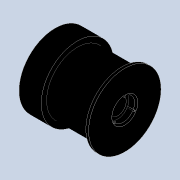
# Autodesk Inventor part: 8mm ID 15mm Deep Idler Pully
Saved by Autodesk Inventor 2022 (Build 260153000, 153)
## iProperties
Created: 2021-10-11
Part Number: 8mm ID 15mm Deep Idler Pully
Material: Generic
Document SubType Name: Modeling
Designer: Coy
Density: 1 g/cm^3
Appearance: Anodized - Black
Author: Coy
Autodesk Inventor part; units mm, degrees
ref_plane "YZ Plane" through (0, 0, 0) normal (1, 0, 0) x (0, 1, 0)
ref_plane "XZ Plane" through (0, 0, 0) normal (0, 1, 0) x (-1, 0, 0)
ref_plane "XY Plane" through (0, 0, 0) normal (0, 0, 1) x (1, 0, 0)
sketch "Sketch1" plane through (0, 0, 0) normal (1, 0, 0) x (0, 1, 0)
  circle A0 centre (0, 0) radius 4
  circle A1 centre (0, 0) radius 13
  dimension "d0" = 8
  dimension "d1" = 26
  constraints: 2 centre point, 2 coincident
  measures "d0" diameter of A0
  measures "d1" diameter of A1
extrude "Extrusion1" add sketch "Sketch1" along normal blind 2.5
sketch "Sketch2" plane through (2.5, 0, 0) normal (1, 0, 0) x (0, 0, -1)
  circle A0 centre (0, 0) radius 3
  circle A1 centre (0, 0) radius 13
  dimension "d4" = 6
  constraints: 2 centre point, 2 coincident
  measures "d4" diameter of A0
extrude "Extrusion2" add sketch "Sketch2" along normal blind 5.5
sketch "Sketch3" plane through (8, 0, 0) normal (1, 0, 0) x (0, 0, -1)
  circle A0 centre (0, 0) radius 3 projected
  circle A1 centre (0, 0) radius 11.08
  dimension "d7" = 22.16
  constraints: 1 centre point, 1 coincident
  measures "d7" diameter of A1
extrude "Extrusion3" add sketch "Sketch3" along normal blind 16
sketch "Sketch4" plane through (24, 0, 0) normal (1, 0, 0) x (0, 0, -1)
  circle A0 centre (0, 0) radius 13 projected
  circle A1 centre (0, 0) radius 3 projected
extrude "Extrusion4" add sketch "Sketch4" along normal blind 1
sketch "Sketch5" plane through (25, 0, 0) normal (1, 0, 0) x (0, 0, -1)
  circle A0 centre (0, 0) radius 4
  dimension "d12" = 8
  constraints: 1 centre point, 1 coincident
  measures "d12" diameter of A0
extrude "Extrusion5" cut sketch "Sketch5" against normal blind 2.5
chamfer "Chamfer1" distance 2.5 angle 2 1 edges at (0, -4, 0) measured on face at (1.6667, 3.9482, -0.6416)
chamfer "Chamfer2" distance 2.5 angle 2 1 edges at (25, 0, 4) measured on face at (23.3333, -0.6416, -3.9482)
sketch "Sketch6" plane through (0, 0, 0) normal (-1, 0, 0) x (0, 0, 1)
  line L0 (0.2, 4.0824) -> (0.2, 3.995)
  line L1 (-0.2, 4.0824) -> (-0.2, 3.995)
  line L2 (0, 0) -> (0, 3.9651) construction
  circle A0 centre (0, 0) radius 4 construction
  arc A1 (-0.2, 4) -> (0.2, 4) centre (0, 4) ccw
  circle A2 centre (0, 0) radius 4.0873 projected
  line L3 (-3.4355, -2.2144) -> (-3.3598, -2.1707)
  arc A3 (-3.3641, -2.1732) -> (-3.5641, -1.8268) centre (-3.4641, -2) ccw
  line L4 (-3.6355, -1.868) -> (-3.5598, -1.8243)
  line L5 (3.6355, -1.868) -> (3.5598, -1.8243)
  arc A4 (3.5641, -1.8268) -> (3.3641, -2.1732) centre (3.4641, -2) ccw
  line L6 (3.4355, -2.2144) -> (3.3598, -2.1707)
  dimension "d21" = 0.2
  dimension "d22" = 0.2
  dimension "d23" = 0.4
  dimension "d26" = 360
  constraints: 14 end point, 11 point on circle, 6 point on line, 3 centre point, 3 vertical, 31 other
  measures "d21" distance between parallel lines of L2 L0
  measures "d22" distance between parallel lines of L2 L1
  measures "d23" diameter of A1
extrude "Extrusion6" add sketch "Sketch6" against normal blind 2.5 contours L0 A1 L1 A2 | A2 L6 A4 L5 | L4 A3 L3 A2
sketch "Sketch7" plane through (25, 0, 0) normal (1, 0, 0) x (0, 0, -1)
  circle A0 centre (0, 0) radius 13 projected
  arc A1 (-0.2, 4.0824) -> (-3.6355, -1.868) centre (0, 0) ccw projected
  line L0 (-3.6355, -1.868) -> (-3.5641, -1.8268) projected
  arc A2 (-3.3641, -2.1732) -> (-3.5641, -1.8268) centre (-3.4641, -2) ccw projected
  line L1 (-3.3641, -2.1732) -> (-3.4355, -2.2144) projected
  arc A3 (-3.4355, -2.2144) -> (3.4355, -2.2144) centre (0, 0) ccw projected
  line L2 (3.4355, -2.2144) -> (3.3641, -2.1732) projected
  arc A4 (3.5641, -1.8268) -> (3.3641, -2.1732) centre (3.4641, -2) ccw projected
  line L3 (3.5641, -1.8268) -> (3.6355, -1.868) projected
  arc A5 (3.6355, -1.868) -> (0.2, 4.0824) centre (0, 0) ccw projected
  line L4 (0.2, 4.0824) -> (0.2, 4) projected
  arc A6 (-0.2, 4) -> (0.2, 4) centre (0, 4) ccw projected
  line L5 (-0.2, 4) -> (-0.2, 4.0824) projected
  circle A7 centre (0, 0) radius 13 projected
  circle A8 centre (0, 0) radius 4.0873 projected
  point P0 (3.4355, -2.2144)
  point P1 (-3.6355, -1.868)
  point P2 (0.2, 4.0824)
  point P3 (-0.2, 4.0824)
extrude "Extrusion7" add sketch "Sketch7" against normal blind 2.5 contours A8 L4 A6 L5 | L0 A2 L1 A8 | L2 A4 L3 A8
fillet "Fillet1" radius 0.6 6 edges at (25, 2.0434, -3.5393) (25, -4.0868, 0) (25, 2.0434, 3.5393) (0, 2.0434, -3.5393) (0, 2.0434, 3.5393) (0, -4.0868, 0)
body "Solid1"
